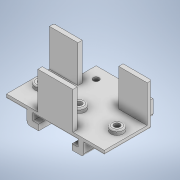
# Autodesk Inventor part: railBracketTop
Saved by Autodesk Inventor 2020 (Build 240168000, 168)
## iProperties
Created: 2020-01-08
Part Number: railBracketTop
Material: Generic
Document SubType Name: Modeling
Designer: PAB
Density: 1 g/cm^3
Appearance: Default
Author: PAB
Autodesk Inventor part; units mm, degrees
ref_plane "YZ Plane" through (0, 0, 0) normal (1, 0, 0) x (0, 1, 0)
ref_plane "XZ Plane" through (0, 0, 0) normal (0, 1, 0) x (-1, 0, 0)
ref_plane "XY Plane" through (0, 0, 0) normal (0, 0, 1) x (1, 0, 0)
sketch "Sketch1" plane through (0, 0, 0) normal (0, 1, 0) x (-1, 0, 0)
  line L0 (20.5, 16.2) -> (-20.5, 16.2)
  line L1 (-20.5, 16.2) -> (-20.5, -16.2)
  line L2 (-20.5, -16.2) -> (20.5, -16.2)
  line L3 (20.5, -16.2) -> (20.5, 16.2)
  point P0 (0, 0)
  dimension "d0" = 41
  dimension "d1" = 32.4
  constraints: 8 end point, 2 parallel, 1 horizontal, 1 perpendicular
  measures "d0" distance of L2.end L1.end
  measures "d1" distance of L1.end L0.end
extrude "Extrusion1" add sketch "Sketch1" along normal blind 3
sketch "Sketch3" plane through (0, 3, 0) normal (0, 1, 0) x (1, 0, 0)
  line L0 (-20.5, -16.2) -> (20.5, -16.2) projected
  line L1 (-20.5, 16.2) -> (-20.5, -16.2) projected
  line L2 (20.5, -16.2) -> (-20.5, -16.2)
  line L3 (-20.5, -16.2) -> (-20.5, -13.2)
  line L4 (-20.5, -13.2) -> (20.5, -13.2)
  line L5 (20.5, -13.2) -> (20.5, -16.2)
  line L6 (20.5, 16.2) -> (-20.5, 16.2) projected
  line L7 (20.5, 16.2) -> (-20.5, 16.2)
  line L8 (-20.5, 16.2) -> (-20.5, 13.2)
  line L9 (-20.5, 13.2) -> (20.5, 13.2)
  line L10 (20.5, 13.2) -> (20.5, 16.2)
  point P0 (0, 0)
  dimension "d8" = 3
  dimension "d9" = 3
  constraints: 16 end point, 4 parallel, 2 horizontal, 2 perpendicular, 2 point on line
  measures "d8" distance of L2.end L3.end
  measures "d9" distance of L8.end L7.end
extrude "Extrusion3" add sketch "Sketch3" along normal blind 25.4
sketch "Sketch4" plane through (20.5, 0, -16.2) normal (0, 0, -1) x (-1, 0, 0)
  line L0 (41, 3) -> (0, 3) projected
  line L1 (0, 28.4) -> (41, 28.4) projected
  line L2 (0, 3) -> (21.5, 3)
  line L3 (21.5, 3) -> (21.5, 28.4)
  line L4 (21.5, 28.4) -> (0, 28.4)
  line L5 (0, 28.4) -> (0, 3)
  point P0 (20.5, 0)
  dimension "d12" = 21.5
  constraints: 8 end point, 2 parallel, 1 horizontal, 1 perpendicular, 1 point on line
  measures "d12" distance of L4.end L3.end
extrude "Extrusion4" cut sketch "Sketch4" against normal blind 3
sketch "Sketch5" plane through (-20.5, 0, 16.2) normal (0, 0, 1) x (1, 0, 0)
  line L0 (41, 28.4) -> (0, 28.4) projected
  line L1 (19.5, 3) -> (41, 3) projected
  line L2 (0, 28.4) -> (21.5, 28.4)
  line L3 (21.5, 28.4) -> (21.5, 3)
  line L4 (21.5, 3) -> (0, 3)
  line L5 (0, 3) -> (0, 28.4)
  point P0 (20.5, 0)
  dimension "d15" = 21.5
  constraints: 8 end point, 2 parallel, 1 horizontal, 1 perpendicular, 1 point on line
  measures "d15" distance of L3.end L4.end
extrude "Extrusion5" cut sketch "Sketch5" against normal blind 3
sketch "Sketch6" plane through (0, 3, 0) normal (0, 1, 0) x (1, 0, 0)
  circle A0 centre (13, 0) radius 4.25
  circle A1 centre (-13, 0) radius 4.25
  line L0 (-20.5, 13.2) -> (-20.5, -16.2) projected
  line L1 (20.5, -13.2) -> (20.5, 16.2) projected
  point P0 (0, 0)
  dimension "d20" = 8.5
  dimension "d21" = 8.5
  dimension "d32" = 26
  dimension "d33" = 7.5
  dimension "d34" = 7.5
  constraints: 2 centre point
  measures "d20" diameter of A0
  measures "d21" diameter of A1
  measures "d32" distance of A0.centre A1.centre
  measures "d33" distance from line of L0 A1.centre
  measures "d34" distance from line of L1 A0.centre
extrude "Extrusion6" add sketch "Sketch6" along normal blind 3
sketch "Sketch9" plane through (20.5, 0, 16.2) normal (1, 0, 0) x (0, 0, -1)
  line L0 (32.4, 0) -> (32.4, 3) projected
  line L1 (32.4, 3) -> (0, 3)
  line L2 (0, 3) -> (0, 0)
  line L3 (0, 0) -> (32.4, 0)
  line L4 (32.4, 0) -> (32.4, 3)
  point P0 (16.2, 0)
  constraints: 8 end point, 2 parallel, 1 horizontal, 1 perpendicular
extrude "Extrusion9" add sketch "Sketch9" along normal blind 26
sketch "Sketch10" plane through (0, 3, 0) normal (0, 1, 0) x (1, 0, 0)
  circle A0 centre (39, 0) radius 4.25
  point P0 (0, 0)
  dimension "d37" = 8.5
  constraints: 1 centre point
  measures "d37" diameter of A0
extrude "Extrusion10" add sketch "Sketch10" along normal blind 3
sketch "Sketch11" plane through (0, 3, 0) normal (0, 1, 0) x (1, 0, 0)
  line L0 (46.5, 16.2) -> (46.5, -16.2) projected
  line L1 (46.5, 16.2) -> (27, 16.2)
  line L2 (27, 16.2) -> (27, 13.2)
  line L3 (27, 13.2) -> (46.5, 13.2)
  line L4 (46.5, 13.2) -> (46.5, 16.2)
  point P0 (0, 0)
  dimension "d40" = 19.5
  dimension "d41" = 3
  constraints: 8 end point, 2 parallel, 1 horizontal, 1 perpendicular
  measures "d40" distance of L3.end L2.end
  measures "d41" distance of L2.end L1.end
extrude "Extrusion11" add sketch "Sketch11" along normal blind 25.4
sketch "Sketch14" plane through (20.5, 3, 13.2) normal (1, 0, 0) x (0, 0, -1)
  line L0 (0, 0) -> (0, 25.4) projected
  line L1 (-3, 0) -> (-3, 25.4) projected
  line L2 (0, 25.4) -> (-3, 25.4)
  line L3 (-3, 25.4) -> (-3, 0)
  line L4 (-3, 0) -> (0, 0)
  line L5 (0, 0) -> (0, 25.4)
  point P0 (13.2, -3)
  constraints: 8 end point, 2 parallel, 1 horizontal, 1 perpendicular
extrude "Extrusion14" add sketch "Sketch14" along normal blind 4.5
fillet "Fillet1" radius 1 3 edges at (-17.25, 6, 0) (8.75, 6, 0) (34.75, 6, 0)
fillet "Fillet2" radius 1 6 edges at (-20.5, 14.2, -16.2) (-20.5, 0, 0) (13, 0, 16.2) (46.5, 0, 0) (46.5, 14.2, -16.2) (13, 0, -16.2)
sketch "Sketch15" plane through (0, 0, 0) normal (0, -1, 0) x (1, 0, 0)
  circle A0 centre (39, 0) radius 4.25 projected
  circle A1 centre (39, 0) radius 2
  circle A2 centre (13, 0) radius 3.25 projected
  circle A3 centre (13, 0) radius 2
  circle A4 centre (-13, 0) radius 3.25 projected
  circle A5 centre (-13, 0) radius 2
  point P0 (0, 0)
  dimension "d54" = 4
  dimension "d55" = 4
  dimension "d56" = 4
  constraints: 3 centre point, 3 coincident
  measures "d54" diameter of A1
  measures "d55" diameter of A3
  measures "d56" diameter of A5
extrude "Extrusion15" cut sketch "Sketch15" against normal blind 10 contours A1 | A3 | A5
sketch "Sketch16" plane through (0, 0, 0) normal (0, -1, 0) x (1, 0, 0)
  circle A0 centre (39, 0) radius 2 projected
  circle A1 centre (39, 0) radius 3
  circle A2 centre (13, 0) radius 2 projected
  circle A3 centre (13, 0) radius 3
  circle A4 centre (-13, 0) radius 2 projected
  circle A5 centre (-13, 0) radius 3
  point P0 (0, 0)
  dimension "d59" = 6
  dimension "d60" = 6
  dimension "d61" = 6
  constraints: 3 centre point, 3 coincident
  measures "d59" diameter of A1
  measures "d60" diameter of A3
  measures "d61" diameter of A5
extrude "Extrusion16" cut sketch "Sketch16" against normal blind 3 contours A0 | A1 | A2 | A3 | A4 | A5
sketch "Sketch17" plane through (0, 0, 0) normal (0, -1, 0) x (1, 0, 0)
  line L0 (46.5, 16.2) -> (-20.5, 16.2) projected
  line L1 (-19.5, -16.2) -> (45.5, -16.2) projected
  line L2 (-2.5, 16.2) -> (-6.5, 16.2)
  line L3 (-6.5, 16.2) -> (-6.5, -16.2)
  line L4 (-6.5, -16.2) -> (-2.5, -16.2)
  line L5 (-2.5, -16.2) -> (-2.5, 16.2)
  line L6 (28.5, 16.2) -> (32.5, 16.2)
  line L7 (32.5, 16.2) -> (32.5, -16.2)
  line L8 (32.5, -16.2) -> (28.5, -16.2)
  line L9 (28.5, -16.2) -> (28.5, 16.2)
  point P0 (0, 0)
  dimension "d64" = 4
  dimension "d65" = 4
  constraints: 16 end point, 4 parallel, 4 point on line, 2 horizontal, 2 perpendicular
  measures "d64" distance of L4.end L3.end
  measures "d65" distance of L7.end L8.end
extrude "Extrusion17" add sketch "Sketch17" along normal blind 8 and the other way blind 2 contours L7 L1 L9 L0 | L5 L1 L3 L0
sketch "Sketch18" plane through (28.5, 0, -15.2) normal (-1, 0, 0) x (0, 0, 1)
  line L0 (31.4, -8) -> (31.4, 1) projected
  line L1 (-1, 1) -> (-1, -8) projected
  line L2 (31.4, -8) -> (-1, -8)
  line L3 (-1, -8) -> (-1, -4)
  line L4 (-1, -4) -> (31.4, -4)
  line L5 (31.4, -4) -> (31.4, -8)
  point P0 (15.2, 0)
  dimension "d70" = 4
  constraints: 8 end point, 2 parallel, 1 horizontal, 1 perpendicular, 1 point on line
  measures "d70" distance of L2.end L3.end
extrude "Extrusion18" add sketch "Sketch18" along normal blind 4
sketch "Sketch19" plane through (-2.5, 0, 15.2) normal (1, 0, 0) x (0, 0, -1)
  line L0 (31.4, -8) -> (-1, -8) projected
  line L1 (-1, -4) -> (31.4, -4) projected
  line L2 (-1, -8) -> (31.4, -8)
  line L3 (31.4, -8) -> (31.4, -4)
  line L4 (31.4, -4) -> (-1, -4)
  line L5 (-1, -4) -> (-1, -8)
  point P0 (15.2, 0)
  constraints: 8 end point, 2 parallel, 1 horizontal, 1 perpendicular
extrude "Extrusion19" add sketch "Sketch19" along normal blind 4
sketch "Sketch20" plane through (-1, 3, -16.2) normal (0, 0, -1) x (-1, 0, 0)
  line L0 (5.5, -2) -> (5.5, -11) projected
  line L1 (-26, 0) -> (-47.5, 0) projected
  line L2 (5.5, -3) -> (-33.5, -3)
  line L3 (-33.5, -3) -> (-33.5, 0)
  line L4 (-33.5, 0) -> (5.5, 0)
  line L5 (5.5, 0) -> (5.5, -3)
  line L6 (5.5, -11) -> (1.5, -11)
  line L7 (1.5, -11) -> (1.5, -3)
  line L8 (1.5, -3) -> (5.5, -3)
  line L9 (5.5, -3) -> (5.5, -11)
  line L10 (-33.5, -2) -> (-33.5, -11) projected
  line L11 (-29.5, -2) -> (-29.5, -7) projected
  line L12 (-33.5, -11) -> (-29.5, -11)
  line L13 (-29.5, -11) -> (-29.5, -3)
  line L14 (-29.5, -3) -> (-33.5, -3)
  line L15 (-33.5, -3) -> (-33.5, -11)
  line L16 (-2.5, -7) -> (1.5, -7)
  line L17 (1.5, -7) -> (1.5, -11)
  line L18 (1.5, -11) -> (-2.5, -11)
  line L19 (-2.5, -11) -> (-2.5, -7)
  line L20 (-29.5, -7) -> (-25.5, -7) projected
  line L21 (-25.5, -7) -> (-29.5, -7)
  line L22 (-29.5, -7) -> (-29.5, -11)
  line L23 (-29.5, -11) -> (-25.5, -11)
  line L24 (-25.5, -11) -> (-25.5, -7)
  point P0 (-1, -3)
  dimension "d75" = 39
  constraints: 40 end point, 10 parallel, 5 horizontal, 5 perpendicular, 5 point on line
  measures "d75" distance of L3.end L4.end
extrude "Extrusion20" add sketch "Sketch20" along normal blind 15 and the other way blind 3
sketch "Sketch21" plane through (24.5, 0, -15.2) normal (-1, 0, 0) x (0, 0, 1)
  line L0 (31.4, -8) -> (-16, -8) projected
  line L1 (-16, -8) -> (-3, -8)
  line L2 (-3, -8) -> (-3, -4)
  line L3 (-3, -4) -> (-16, -4)
  line L4 (-16, -4) -> (-16, -8)
  point P0 (15.2, 0)
  dimension "d80" = 13
  dimension "d81" = 4
  constraints: 8 end point, 2 parallel, 1 horizontal, 1 perpendicular
  measures "d80" distance of L3.end L2.end
  measures "d81" distance of L2.end L1.end
extrude "Extrusion21" add sketch "Sketch21" along normal blind 4
sketch "Sketch22" plane through (1.5, 0, 15.2) normal (1, 0, 0) x (0, 0, -1)
  line L0 (46.4, 3) -> (46.4, -8) projected
  line L1 (-1, -4) -> (33.4, -4) projected
  line L2 (46.4, -8) -> (33.4, -8)
  line L3 (33.4, -8) -> (33.4, -4)
  line L4 (33.4, -4) -> (46.4, -4)
  line L5 (46.4, -4) -> (46.4, -8)
  point P0 (15.2, 0)
  dimension "d84" = 4
  constraints: 8 end point, 2 parallel, 1 horizontal, 1 perpendicular
  measures "d84" distance of L2.end L1.end
extrude "Extrusion22" add sketch "Sketch22" along normal blind 4
sketch "Sketch23" plane through (0, -8, 0) normal (0, -1, 0) x (1, 0, 0)
  circle A0 centre (1.5, -23.2) radius 2
  circle A1 centre (24.5, -23.2) radius 2
  point P0 (0, 0)
  dimension "d87" = 4
  dimension "d88" = 4
  constraints: 2 centre point
  measures "d87" diameter of A0
  measures "d88" diameter of A1
extrude "Extrusion23" cut sketch "Sketch23" against normal blind 20
fillet "Fillet3" radius 2 2 edges at (-6.5, -8, -7.5) (32.5, -8, -7.5)
body "Solid1"
